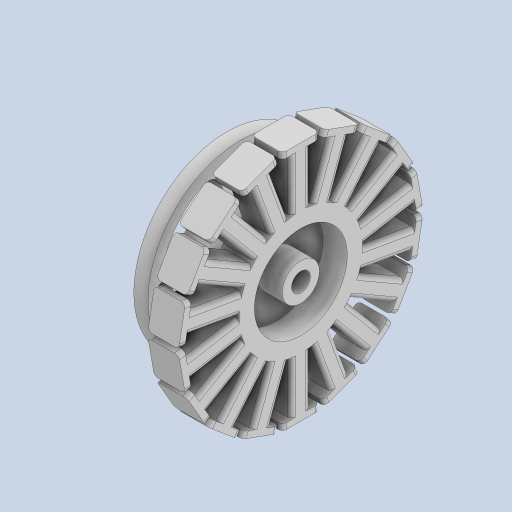
# Autodesk Inventor part: mot_4006_base
Saved by Autodesk Inventor 2023 (Build 270158000, 158)
## iProperties
Created: 2022-10-31
Part Number: mot_4006_base
Material: Generic
Document SubType Name: Modeling
Designer: Shuang Peng
Density: 1 g/cm^3
Appearance: Default
Author: Shuang Peng
Autodesk Inventor part; units mm, degrees
ref_plane "YZ Plane" through (0, 0, 0) normal (1, 0, 0) x (0, 1, 0)
ref_plane "XZ Plane" through (0, 0, 0) normal (0, 1, 0) x (-1, 0, 0)
ref_plane "XY Plane" through (0, 0, 0) normal (0, 0, 1) x (1, 0, 0)
sketch "Sketch1" plane through (0, 0, 0) normal (0, 1, 0) x (-1, 0, 0)
  line L0 (0, 0) -> (170.5593, 0) construction
  line L1 (170.5593, 0) -> (170.5593, -169.2892) construction
  line L2 (170.5593, -169.2892) -> (0, -169.2892) construction
  line L3 (0, -169.2892) -> (0, 0) construction
  line L4 (4.2, 15) -> (4.2, -15)
  line L5 (4.2, 0) -> (6.5, 0)
  line L6 (6.5, 0) -> (6.5, 15)
  line L7 (6.5, 15) -> (4.2, 15)
  line L8 (4.2, 0) -> (0.5, 0)
  line L9 (0.5, 0) -> (0.5, 8)
  line L10 (0.5, 8) -> (4.2, 8)
  line L11 (6.5, 0) -> (6.5, 2)
  line L12 (6.5, 2) -> (6.9, 2)
  line L13 (6.9, 2) -> (6.9, 1.62)
  line L14 (6.9, 1.62) -> (7.4, 1.62)
  line L15 (7.4, 1.62) -> (7.4, 2)
  line L16 (7.4, 2) -> (9, 2)
  line L17 (9, 2) -> (9, 0)
  line L18 (9, 0) -> (6.5, 0)
  line L19 (0.5, 0) -> (-0.5, 0)
  line L20 (-0.5, 0) -> (-0.5, 8)
  line L21 (-0.5, 8) -> (0.5, 8)
  dimension "d52" = 30
  dimension "d77" = 2.3
  dimension "d78" = 15
  dimension "d79" = 3.7
  dimension "d80" = 8
  dimension "d81" = 2
  dimension "d82" = 0.4
  dimension "d83" = 0.38
  dimension "d84" = 0.5
  dimension "d85" = 0.38
  dimension "d86" = 1.6
  dimension "d87" = 2
  dimension "d88" = 1
  constraints: 36 end point, 6 vertical, 5 perpendicular, 3 horizontal, 2 midpoint, 2 point on line, 1 coincident, 1 parallel, 2 other
  measures "d52" distance of L4.start L4.end
  measures "d77" distance of L5.start L5.end
  measures "d78" distance of L5.end L6.end
  measures "d79" distance of L5.start L8.end
  measures "d80" distance of L8.end L9.end
  measures "d81" distance of L5.end L11.end
  measures "d82" distance of L11.end L12.end
  measures "d83" distance of L12.end L13.end
  measures "d84" distance of L13.end L14.end
  measures "d85" distance of L14.end L15.end
  measures "d86" distance of L15.end L16.end
  measures "d87" distance of L16.end L17.end
  measures "d88" distance of L8.end L19.end
revolve "Revolution1" add sketch "Sketch1" angle 360 about axis through (0, 0, 0) along (-1, 0, 0)
sketch "Sketch2" plane through (-6.5, 0, 0) normal (-1, 0, 0) x (0, 0, 1)
  circle A0 centre (0, 0) radius 2 projected
  line L0 (0, 0) -> (-12.5, 0)
  circle A1 centre (-12.5, 0) radius 1.5
  dimension "d90" = 12.5
  dimension "d91" = 3
  constraints: 2 end point, 1 centre point, 1 coincident, 1 horizontal
  measures "d90" distance of L0.start L0.end
  measures "d91" diameter of A1
extrude "Extrusion1" cut sketch "Sketch2" against normal blind 10 contours A1
pattern_circular "Circular Pattern1" count 4 over 360 about axis through (-5.35, 0, 0) along (-1, 0, 0) of "Extrusion1"
sketch "Sketch3" plane through (-6.5, 0, 0) normal (-1, 0, 0) x (0, 0, 1)
  circle A0 centre (0, 12.5) radius 1.5 projected
  circle A1 centre (12.5, 0) radius 1.5 projected
  circle A2 centre (0, -12.5) radius 1.5 projected
  circle A3 centre (-12.5, 0) radius 1.5 projected
  circle A4 centre (0, 0) radius 15 projected
  circle A5 centre (0, 0) radius 2 projected
  circle A6 centre (0, 0) radius 2 projected
  circle A7 centre (0, 0) radius 13.25
  line L0 (-31.1051, 42.2075) -> (134.1997, 72.6613) construction
  line L1 (134.1997, 72.6613) -> (164.4267, -91.4124) construction
  line L2 (164.4267, -91.4124) -> (-0.878, -121.8662) construction
  line L3 (-0.878, -121.8662) -> (-31.1051, 42.2075) construction
  circle A8 centre (0, 0) radius 8
  circle A9 centre (0, 0) radius 8 projected
  circle A10 centre (0, -12.5) radius 1.5 projected
  line L4 (0, -12.5) -> (-12.5, 0)
  line L5 (0, 0) -> (-6.25, -6.25)
  line L6 (0, 0) -> (-12.671, -3.8739)
  line L7 (0, 0) -> (13.25, 0) construction
  line L8 (0, 0) -> (-3.8739, -12.671)
  point P0 (-2.339, -7.6504)
  point P1 (-7.6504, -2.339)
  dimension "d97" = 26.5
  dimension "d122" = 0
  dimension "d123" = 13.25
  dimension "d124" = 163
  dimension "d125" = 28
  constraints: 10 end point, 2 coincident, 1 centre point, 1 equal length, 1 horizontal, 1 midpoint, 5 other
  measures "d122" radial gap between concentric circles of A9 A8
  measures "d123" distance of L5.start L6.end
  measures "d124" angle of L6 L7
  measures "d125" angle of L5 L8
extrude "Extrusion2" cut sketch "Sketch3" against normal blind 10 contours L6 L4 L8 A7 | L6 A8 L5 L4 | L5 A8 L8 L4
fillet "Fillet1" radius 2.2 4 edges at (-5.35, -12.671, -3.8739) (-5.35, -3.8739, -12.671) (-5.35, -2.339, -7.6504) (-5.35, -7.6504, -2.339)
pattern_circular "Circular Pattern2" count 4 over 360 about axis through (-5.35, 0, 0) along (-1, 0, 0) of "Extrusion2", "Fillet1"
sketch "Sketch4" plane through (0.5, 0, 0) normal (1, 0, 0) x (0, 0, -1)
  circle A0 centre (0, 0) radius 2 projected
  circle A1 centre (0, 0) radius 19.5
  line L0 (0, 0) -> (0, 19.5)
  line L1 (0, 0) -> (0, 19)
  line L2 (-3, 19.5) -> (3, 19.5)
  line L3 (3, 19.5) -> (3, 18.5)
  line L4 (3, 18.5) -> (-3, 18.5)
  line L5 (-3, 18.5) -> (-3, 19.5)
  line L6 (-3, 19.5) -> (3, 18.5) construction
  line L7 (3, 19.5) -> (-3, 18.5) construction
  line L8 (-1.5, 0.5) -> (1.5, 0.5)
  line L9 (1.5, 0.5) -> (1.5, 18.5)
  line L10 (1.5, 18.5) -> (-1.5, 18.5)
  line L11 (-1.5, 18.5) -> (-1.5, 0.5)
  line L12 (-1.5, 0.5) -> (1.5, 18.5) construction
  line L13 (1.5, 0.5) -> (-1.5, 18.5) construction
  point P0 (0, 0)
  point P1 (0, 9.5)
  dimension "d132" = 39
  dimension "d133" = 19
  dimension "d134" = 6
  dimension "d135" = 1
  dimension "d136" = 3
  dimension "d137" = 18
  constraints: 28 end point, 5 midpoint, 4 parallel, 3 perpendicular, 1 coincident, 1 horizontal, 1 point on line, 1 vertical, 1 vertical alignment, 2 other
  measures "d133" distance of L0.start L1.end
  measures "d134" distance of L2.start L2.end
  measures "d135" distance of L2.end L3.end
  measures "d136" distance of L8.start L8.end
  measures "d137" distance of L9.end L8.end
extrude "Extrusion3" add sketch "Sketch4" along normal blind 5 contours L9 L8 L0 A0 | A0 L0 L4 L9 | L11 L4 L0 A0 | A0 L0 L8 L11 | L4 L0 A1 L3 | L4 L5 A1 L0 | A1 L2 L3 | L5 L2 A1
pattern_circular "Circular Pattern3" count 18 over 360 about axis through (-1.85, 0, 0) along (-1, 0, 0) of "Extrusion3"
sketch "Sketch5" plane through (5.5, 0, 0) normal (1, 0, 0) x (0, 0, -1)
  circle A0 centre (0, 0) radius 2 projected
  circle A1 centre (0, 0) radius 10
  point P0 (0, 0)
  dimension "d143" = 20
  constraints: 1 centre point, 1 coincident
  measures "d143" diameter of A1
extrude "Extrusion4" add sketch "Sketch5" against normal up to surface (5 mm away)
fillet "Fillet2" radius 0.7 4 edges at (0.5, 5.7977, -13.0419) (0.5, 8.3958, -11.5419) (5.5, 5.7977, -13.0419) (5.5, 8.3958, -11.5419)
pattern_circular "Circular Pattern4" count 18 over 360 about axis through (5.5, 0, 0) along (-1, 0, 0) of "Fillet2"
fillet "Fillet3" radius 0.7 4 edges at (5.5, 12.6265, 14.5111) (5.5, 16.4832, 9.9148) (0.5, 16.4832, 9.9148) (0.5, 12.6265, 14.5111)
pattern_circular "Circular Pattern5" count 18 over 360 about axis through (-5.35, 0, 0) along (-1, 0, 0) of "Fillet3"
sketch "Sketch6" plane through (5.5, 0, 0) normal (1, 0, 0) x (0, 0, -1)
  line L0 (-15.7375, 11.7419) -> (-14.8715, 11.2419) projected
  line L1 (-15.7375, 11.7419) -> (-18.0375, 7.7581) projected
  line L2 (-17.1715, 7.2581) -> (-18.0375, 7.7581) projected
  line L3 (-17.1715, 7.2581) -> (-16.4215, 8.5572) projected
  line L4 (-9.0325, 4.2912) -> (-16.4215, 8.5572) projected
  arc A0 (-9.0325, 4.2912) -> (-9.6776, 2.5188) centre (0, 0) ccw projected
  line L5 (-18.08, 4.0003) -> (-9.6776, 2.5188) projected
  line L6 (-18.08, 4.0003) -> (-17.8196, 5.4775) projected
  line L7 (-18.8044, 5.6512) -> (-17.8196, 5.4775) projected
  line L8 (-18.8044, 5.6512) -> (-19.6031, 1.1211) projected
  line L9 (-18.6183, 0.9474) -> (-19.6031, 1.1211) projected
  line L10 (-18.6183, 0.9474) -> (-18.3579, 2.4246) projected
  line L11 (-9.9554, 0.9431) -> (-18.3579, 2.4246) projected
  arc A1 (-9.9554, 0.9431) -> (-9.9554, -0.9431) centre (0, 0) ccw projected
  line L12 (-18.3579, -2.4246) -> (-9.9554, -0.9431) projected
  line L13 (-18.3579, -2.4246) -> (-18.6183, -0.9474) projected
  line L14 (-19.6031, -1.1211) -> (-18.6183, -0.9474) projected
  line L15 (-19.6031, -1.1211) -> (-18.8044, -5.6512) projected
  line L16 (-17.8196, -5.4775) -> (-18.8044, -5.6512) projected
  line L17 (-17.8196, -5.4775) -> (-18.08, -4.0003) projected
  line L18 (-9.6776, -2.5188) -> (-18.08, -4.0003) projected
  arc A2 (-9.6776, -2.5188) -> (-9.0325, -4.2912) centre (0, 0) ccw projected
  line L19 (-16.4215, -8.5572) -> (-9.0325, -4.2912) projected
  line L20 (-16.4215, -8.5572) -> (-17.1715, -7.2581) projected
  line L21 (-18.0375, -7.7581) -> (-17.1715, -7.2581) projected
  line L22 (-18.0375, -7.7581) -> (-15.7375, -11.7419) projected
  line L23 (-14.8715, -11.2419) -> (-15.7375, -11.7419) projected
  line L24 (-14.8715, -11.2419) -> (-15.6215, -9.9428) projected
  line L25 (-8.2325, -5.6768) -> (-15.6215, -9.9428) projected
  arc A3 (-8.2325, -5.6768) -> (-7.0201, -7.1217) centre (0, 0) ccw projected
  line L26 (-12.5044, -13.6576) -> (-7.0201, -7.1217) projected
  line L27 (-12.5044, -13.6576) -> (-13.6535, -12.6934) projected
  line L28 (-14.2963, -13.4595) -> (-13.6535, -12.6934) projected
  line L29 (-14.2963, -13.4595) -> (-10.7725, -16.4163) projected
  line L30 (-10.1297, -15.6502) -> (-10.7725, -16.4163) projected
  line L31 (-10.1297, -15.6502) -> (-11.2787, -14.6861) projected
  line L32 (-5.7944, -8.1501) -> (-11.2787, -14.6861) projected
  arc A4 (-5.7944, -8.1501) -> (-4.161, -9.0932) centre (0, 0) ccw projected
  line L33 (-7.0791, -17.1107) -> (-4.161, -9.0932) projected
  line L34 (-7.0791, -17.1107) -> (-8.4887, -16.5977) projected
  line L35 (-8.8307, -17.5374) -> (-8.4887, -16.5977) projected
  line L36 (-8.8307, -17.5374) -> (-4.5081, -19.1107) projected
  line L37 (-4.1661, -18.171) -> (-4.5081, -19.1107) projected
  line L38 (-4.1661, -18.171) -> (-5.5756, -17.6579) projected
  line L39 (-2.6575, -9.6404) -> (-5.5756, -17.6579) projected
  arc A5 (-2.6575, -9.6404) -> (-0.8, -9.9679) centre (0, 0) ccw projected
  line L40 (-0.8, -18.5) -> (-0.8, -9.9679) projected
  line L41 (-0.8, -18.5) -> (-2.3, -18.5) projected
  line L42 (-2.3, -19.5) -> (-2.3, -18.5) projected
  line L43 (-2.3, -19.5) -> (2.3, -19.5) projected
  line L44 (2.3, -18.5) -> (2.3, -19.5) projected
  line L45 (2.3, -18.5) -> (0.8, -18.5) projected
  line L46 (0.8, -9.9679) -> (0.8, -18.5) projected
  arc A6 (0.8, -9.9679) -> (2.6575, -9.6404) centre (0, 0) ccw projected
  line L47 (5.5756, -17.6579) -> (2.6575, -9.6404) projected
  line L48 (5.5756, -17.6579) -> (4.1661, -18.171) projected
  line L49 (4.5081, -19.1107) -> (4.1661, -18.171) projected
  line L50 (4.5081, -19.1107) -> (8.8307, -17.5374) projected
  line L51 (8.4887, -16.5977) -> (8.8307, -17.5374) projected
  line L52 (8.4887, -16.5977) -> (7.0791, -17.1107) projected
  line L53 (4.161, -9.0932) -> (7.0791, -17.1107) projected
  arc A7 (4.161, -9.0932) -> (5.7944, -8.1501) centre (0, 0) ccw projected
  line L54 (11.2787, -14.6861) -> (5.7944, -8.1501) projected
  line L55 (11.2787, -14.6861) -> (10.1297, -15.6502) projected
  line L56 (10.7725, -16.4163) -> (10.1297, -15.6502) projected
  line L57 (10.7725, -16.4163) -> (14.2963, -13.4595) projected
  line L58 (13.6535, -12.6934) -> (14.2963, -13.4595) projected
  line L59 (13.6535, -12.6934) -> (12.5044, -13.6576) projected
  line L60 (7.0201, -7.1217) -> (12.5044, -13.6576) projected
  arc A8 (7.0201, -7.1217) -> (8.2325, -5.6768) centre (0, 0) ccw projected
  line L61 (15.6215, -9.9428) -> (8.2325, -5.6768) projected
  line L62 (15.6215, -9.9428) -> (14.8715, -11.2419) projected
  line L63 (15.7375, -11.7419) -> (14.8715, -11.2419) projected
  line L64 (15.7375, -11.7419) -> (18.0375, -7.7581) projected
  line L65 (17.1715, -7.2581) -> (18.0375, -7.7581) projected
  line L66 (17.1715, -7.2581) -> (16.4215, -8.5572) projected
  line L67 (9.0325, -4.2912) -> (16.4215, -8.5572) projected
  arc A9 (9.0325, -4.2912) -> (9.6776, -2.5188) centre (0, 0) ccw projected
  line L68 (18.08, -4.0003) -> (9.6776, -2.5188) projected
  line L69 (18.08, -4.0003) -> (17.8196, -5.4775) projected
  line L70 (18.8044, -5.6512) -> (17.8196, -5.4775) projected
  line L71 (18.8044, -5.6512) -> (19.6031, -1.1211) projected
  line L72 (18.6183, -0.9474) -> (19.6031, -1.1211) projected
  line L73 (18.6183, -0.9474) -> (18.3579, -2.4246) projected
  line L74 (9.9554, -0.9431) -> (18.3579, -2.4246) projected
  arc A10 (9.9554, -0.9431) -> (9.9554, 0.9431) centre (0, 0) ccw projected
  line L75 (18.3579, 2.4246) -> (9.9554, 0.9431) projected
  line L76 (18.3579, 2.4246) -> (18.6183, 0.9474) projected
  line L77 (19.6031, 1.1211) -> (18.6183, 0.9474) projected
  line L78 (19.6031, 1.1211) -> (18.8044, 5.6512) projected
  line L79 (17.8196, 5.4775) -> (18.8044, 5.6512) projected
  line L80 (17.8196, 5.4775) -> (18.08, 4.0003) projected
  line L81 (9.6776, 2.5188) -> (18.08, 4.0003) projected
  arc A11 (9.6776, 2.5188) -> (9.0325, 4.2912) centre (0, 0) ccw projected
  line L82 (16.4215, 8.5572) -> (9.0325, 4.2912) projected
  line L83 (16.4215, 8.5572) -> (17.1715, 7.2581) projected
  line L84 (18.0375, 7.7581) -> (17.1715, 7.2581) projected
  line L85 (18.0375, 7.7581) -> (15.7375, 11.7419) projected
  line L86 (14.8715, 11.2419) -> (15.7375, 11.7419) projected
  line L87 (14.8715, 11.2419) -> (15.6215, 9.9428) projected
  line L88 (8.2325, 5.6768) -> (15.6215, 9.9428) projected
  arc A12 (8.2325, 5.6768) -> (7.0201, 7.1217) centre (0, 0) ccw projected
  line L89 (12.5044, 13.6576) -> (7.0201, 7.1217) projected
  line L90 (12.5044, 13.6576) -> (13.6535, 12.6934) projected
  line L91 (14.2963, 13.4595) -> (13.6535, 12.6934) projected
  line L92 (14.2963, 13.4595) -> (10.7725, 16.4163) projected
  line L93 (10.1297, 15.6502) -> (10.7725, 16.4163) projected
  line L94 (10.1297, 15.6502) -> (11.2787, 14.6861) projected
  line L95 (5.7944, 8.1501) -> (11.2787, 14.6861) projected
  arc A13 (5.7944, 8.1501) -> (4.161, 9.0932) centre (0, 0) ccw projected
  line L96 (7.0791, 17.1107) -> (4.161, 9.0932) projected
  line L97 (7.0791, 17.1107) -> (8.4887, 16.5977) projected
  line L98 (8.8307, 17.5374) -> (8.4887, 16.5977) projected
  line L99 (8.8307, 17.5374) -> (4.5081, 19.1107) projected
  line L100 (4.1661, 18.171) -> (4.5081, 19.1107) projected
  line L101 (4.1661, 18.171) -> (5.5756, 17.6579) projected
  line L102 (2.6575, 9.6404) -> (5.5756, 17.6579) projected
  arc A14 (2.6575, 9.6404) -> (0.8, 9.9679) centre (0, 0) ccw projected
  line L103 (0.8, 18.5) -> (0.8, 9.9679) projected
  line L104 (0.8, 18.5) -> (2.3, 18.5) projected
  line L105 (2.3, 19.5) -> (2.3, 18.5) projected
  line L106 (2.3, 19.5) -> (-2.3, 19.5) projected
  line L107 (-2.3, 18.5) -> (-2.3, 19.5) projected
  line L108 (-2.3, 18.5) -> (-0.8, 18.5) projected
  line L109 (-0.8, 9.9679) -> (-0.8, 18.5) projected
  arc A15 (-0.8, 9.9679) -> (-2.6575, 9.6404) centre (0, 0) ccw projected
  line L110 (-5.5756, 17.6579) -> (-2.6575, 9.6404) projected
  line L111 (-5.5756, 17.6579) -> (-4.1661, 18.171) projected
  line L112 (-4.5081, 19.1107) -> (-4.1661, 18.171) projected
  line L113 (-4.5081, 19.1107) -> (-8.8307, 17.5374) projected
  line L114 (-8.4887, 16.5977) -> (-8.8307, 17.5374) projected
  line L115 (-8.4887, 16.5977) -> (-7.0791, 17.1107) projected
  line L116 (-4.161, 9.0932) -> (-7.0791, 17.1107) projected
  arc A16 (-4.161, 9.0932) -> (-5.7944, 8.1501) centre (0, 0) ccw projected
  line L117 (-11.2787, 14.6861) -> (-5.7944, 8.1501) projected
  line L118 (-11.2787, 14.6861) -> (-10.1297, 15.6502) projected
  line L119 (-10.7725, 16.4163) -> (-10.1297, 15.6502) projected
  line L120 (-10.7725, 16.4163) -> (-14.2963, 13.4595) projected
  line L121 (-13.6535, 12.6934) -> (-14.2963, 13.4595) projected
  line L122 (-13.6535, 12.6934) -> (-12.5044, 13.6576) projected
  line L123 (-7.0201, 7.1217) -> (-12.5044, 13.6576) projected
  arc A17 (-7.0201, 7.1217) -> (-8.2325, 5.6768) centre (0, 0) ccw projected
  line L124 (-15.6215, 9.9428) -> (-8.2325, 5.6768) projected
  line L125 (-15.6215, 9.9428) -> (-14.8715, 11.2419) projected
  line L126 (-0.0882, 0.5) -> (0.0882, 0.5) projected
  line L127 (0.0882, 0.5) -> (0.2539, 0.4397) projected
  line L128 (0.2539, 0.4397) -> (0.3889, 0.3264) projected
  line L129 (0.3889, 0.3264) -> (0.4771, 0.1736) projected
  line L130 (0.4771, 0.1736) -> (0.5077, 0) projected
  line L131 (0.5077, 0) -> (0.4771, -0.1736) projected
  line L132 (0.4771, -0.1736) -> (0.3889, -0.3264) projected
  line L133 (0.3889, -0.3264) -> (0.2539, -0.4397) projected
  line L134 (0.2539, -0.4397) -> (0.0882, -0.5) projected
  line L135 (0.0882, -0.5) -> (-0.0882, -0.5) projected
  line L136 (-0.0882, -0.5) -> (-0.2539, -0.4397) projected
  line L137 (-0.2539, -0.4397) -> (-0.3889, -0.3264) projected
  line L138 (-0.3889, -0.3264) -> (-0.4771, -0.1736) projected
  line L139 (-0.4771, -0.1736) -> (-0.5077, 0) projected
  line L140 (-0.5077, 0) -> (-0.4771, 0.1736) projected
  line L141 (-0.4771, 0.1736) -> (-0.3889, 0.3264) projected
  line L142 (-0.3889, 0.3264) -> (-0.2539, 0.4397) projected
  line L143 (-0.2539, 0.4397) -> (-0.0882, 0.5) projected
  circle A18 centre (0, 0) radius 1.5
  point P0 (0, 0)
  dimension "d154" = 3
  constraints: 1 centre point, 1 coincident
  measures "d154" diameter of A18
extrude "Extrusion5" cut sketch "Sketch6" against normal blind 8 contours L126 L127 L128 L129 L130 L131 L132 L133 L134 L135 L136 L137 L138 L139 L140 L141 L142 L143 | A18
sketch "Sketch7" plane through (5.5, 0, 0) normal (1, 0, 0) x (0, 0, -1)
  circle A0 centre (0, 0) radius 3
  circle A1 centre (0, 0) radius 7.5
  dimension "d157" = 6
  dimension "d158" = 15
  constraints: 2 centre point, 2 coincident
  measures "d157" diameter of A0
  measures "d158" diameter of A1
extrude "Extrusion6" cut sketch "Sketch7" against normal blind 4
body "Solid1"
